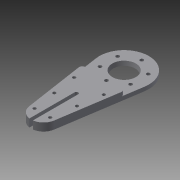
# Autodesk Inventor part: JointD0_2nd
Saved by Autodesk Inventor 2013 (Build 170138000, 138)
## iProperties
Created: 2013-02-07
Part Number: JointD0_2nd
Document SubType Name: Modeling
Designer: JohnHenry
Density: 1 g/cm^3
Material: 一般
Author: JohnHenry
Autodesk Inventor part; units mm, degrees
ref_plane "YZ Plane" through (0, 0, 0) normal (1, 0, 0) x (0, 1, 0)
ref_plane "XZ Plane" through (0, 0, 0) normal (0, 1, 0) x (-1, 0, 0)
ref_plane "XY Plane" through (0, 0, 0) normal (0, 0, 1) x (1, 0, 0)
sketch "スケッチ1" plane through (0, 0, 0) normal (0, 0, 1) x (1, 0, 0)
  circle A0 centre (0, 0) radius 15.75
  line L0 (0, -104.25) -> (0, 0)
  line L1 (0, -104.25) -> (-15.5692, -2.3795)
  line L2 (0, -104.25) -> (15.5692, -2.3795)
  point P0 (0, 15.75)
  point P1 (0, 15.75)
  dimension "d0" = 31.5
  dimension "d1" = 120
  constraints: 6 end point, 3 point on circle, 2 coincident, 2 tangent, 1 centre point, 1 vertical
  measures "d0" diameter of A0
  measures "d1" distance of L0.start A0.start
extrude "押し出し1" add sketch "スケッチ1" along normal blind 5
fillet "フィレット1" radius 8 1 edges at (0, -104.25, 2.5)
sketch "スケッチ2" plane through (0, 0, 5) normal (0, 0, 1) x (1, 0, 0)
  arc A0 (15.5692, -2.3795) -> (-15.5692, -2.3795) centre (0, 0) ccw projected
  constraints: 1 coincident
hole "Hole1" at (0, 0, 5) direction (0, 0, -1) diameter 13 depth 8 tip angle 118
sketch "スケッチ3" plane through (0, 0, 5) normal (0, 0, 1) x (1, 0, 0)
  arc A0 (-7.9082, -52.5063) -> (7.9082, -52.5063) centre (0, -51.2976) ccw projected
  line L0 (-1.1, -29.2976) -> (1.1, -29.2976)
  line L1 (1.1, -29.2976) -> (1.1, -59.2976)
  line L2 (1.1, -59.2976) -> (-1.1, -59.2976)
  line L3 (-1.1, -59.2976) -> (-1.1, -29.2976)
  dimension "d12" = 2.2
  dimension "d13" = 1.1
  dimension "d14" = 30
  dimension "d15" = 0
  constraints: 8 end point, 2 parallel, 1 horizontal, 1 perpendicular
  measures "d12" distance of L0.start L0.end
  measures "d13" distance from line of L1 A0.centre
  measures "d14" distance of L0.end L1.end
  measures "d15" distance edge to line of A0 L2
extrude "押し出し2" cut sketch "スケッチ3" against normal through all
fillet "フィレット2" radius 1 2 edges at (-1.1, -29.2976, 2.5) (1.1, -29.2976, 2.5)
sketch "スケッチ4" plane through (0, 0, 5) normal (0, 0, 1) x (1, 0, 0)
  circle A0 centre (0, 0) radius 11.25
  point P0 (0, 11.25)
  point P1 (-9.7428, 5.625)
  point P2 (-9.7428, -5.625)
  point P3 (0, -11.25)
  point P4 (9.7428, -5.625)
  point P5 (9.7428, 5.625)
  dimension "d22" = 22.5
  dimension "d25" = 360
  constraints: 1 vertical alignment, 9 other
hole "Hole2" at (0, 11.25, 5) at (-9.7428, 5.625, 5) at (-9.7428, -5.625, 5) at (0, -11.25, 5) at (9.7428, -5.625, 5) at (9.7428, 5.625, 5) direction (0, 0, -1) diameter 2.2 depth 8 tip angle 118
sketch "スケッチ5" plane through (0, 0, 5) normal (0, 0, 1) x (1, 0, 0)
  circle A0 centre (9.7428, 5.625) radius 1.1 projected
  circle A1 centre (9.7428, -5.625) radius 1.1 projected
  circle A2 centre (0, -11.25) radius 1.1 projected
  circle A3 centre (-9.7428, -5.625) radius 1.1 projected
  circle A4 centre (-9.7428, 5.625) radius 1.1 projected
  circle A5 centre (0, 11.25) radius 1.1 projected
  circle A6 centre (0, 0) radius 7.5 projected
  circle A7 centre (0, 0) radius 17
  dimension "d34" = 34
  constraints: 1 centre point
  measures "d34" diameter of A7
extrude "押し出し3" cut sketch "スケッチ5" against normal blind 2.5 contours A6 | A7
sketch "スケッチ6" plane through (0, 0, 0) normal (0, 0, -1) x (-1, 0, 0)
  circle A0 centre (-9.7428, 5.625) radius 1.1 projected
  circle A1 centre (-9.7428, -5.625) radius 1.1 projected
  circle A2 centre (0, -11.25) radius 1.1 projected
  circle A3 centre (9.7428, -5.625) radius 1.1 projected
  circle A4 centre (9.7428, 5.625) radius 1.1 projected
  circle A5 centre (0, 11.25) radius 1.1 projected
  line L0 (1.1, -30.2976) -> (1.1, -59.2216) projected
  arc A6 (1.1, -59.2216) -> (7.9082, -52.5063) centre (0, -51.2976) ccw projected
  line L1 (15.5692, -2.3795) -> (7.9082, -52.5063) projected
  arc A7 (15.5692, -2.3795) -> (-15.5692, -2.3795) centre (0, 0) ccw projected
  line L2 (-7.9082, -52.5063) -> (-15.5692, -2.3795) projected
  arc A8 (-7.9082, -52.5063) -> (-1.1, -59.2216) centre (0, -51.2976) ccw projected
  line L3 (-1.1, -59.2216) -> (-1.1, -30.2976) projected
  arc A9 (-0.1, -29.2976) -> (-1.1, -30.2976) centre (-0.1, -30.2976) ccw projected
  line L4 (-0.1, -29.2976) -> (0.1, -29.2976) projected
  arc A10 (1.1, -30.2976) -> (0.1, -29.2976) centre (0.1, -30.2976) ccw projected
  circle A11 centre (0, 0) radius 6.5 projected
extrude "押し出し4" add sketch "スケッチ6" along normal blind 2.5
chamfer "面取り2" distance 5 distance2 1 1 edges at (0, 6.5, 2.5) measured on face at (0, 6.5, 2)
sketch "スケッチ7" plane through (0, 0, -2.5) normal (0, 0, -1) x (-1, 0, 0)
  circle A0 centre (0, 0) radius 6.5 projected
  circle A1 centre (0, 11.25) radius 1.1 projected
  circle A2 centre (9.7428, 5.625) radius 1.1 projected
  circle A3 centre (9.7428, -5.625) radius 1.1 projected
  circle A4 centre (0, -11.25) radius 1.1 projected
  circle A5 centre (-9.7428, -5.625) radius 1.1 projected
  circle A6 centre (-9.7428, 5.625) radius 1.1 projected
  arc A7 (1.1, -30.2976) -> (0.1, -29.2976) centre (0.1, -30.2976) ccw projected
  line L0 (1.1, -59.2216) -> (1.1, -30.2976) projected
  arc A8 (1.1, -59.2216) -> (7.9082, -52.5063) centre (0, -51.2976) ccw projected
  line L1 (15.5692, -2.3795) -> (7.9082, -52.5063) projected
  arc A9 (15.5692, -2.3795) -> (-15.5692, -2.3795) centre (0, 0) ccw projected
  line L2 (-7.9082, -52.5063) -> (-15.5692, -2.3795) projected
  arc A10 (-7.9082, -52.5063) -> (-1.1, -59.2216) centre (0, -51.2976) ccw projected
  line L3 (-1.1, -30.2976) -> (-1.1, -59.2216) projected
  arc A11 (-0.1, -29.2976) -> (-1.1, -30.2976) centre (-0.1, -30.2976) ccw projected
  line L4 (0.1, -29.2976) -> (-0.1, -29.2976) projected
extrude "押し出し5" cut sketch "スケッチ7" against normal blind 2.5
fillet "フィレット3" radius 2 2 edges at (-14.6026, -8.7043, 3.75) (14.6026, -8.7043, 3.75)
sketch "スケッチ8" plane through (0, 0, 5) normal (0, 0, 1) x (1, 0, 0)
  line L0 (-7.9082, -52.5063) -> (-13.5882, -15.3415) projected
  line L1 (-0.1, -29.2976) -> (0.1, -29.2976) projected
  arc A0 (1.1, -59.2216) -> (7.9082, -52.5063) centre (0, -51.2976) ccw projected
  circle A1 centre (0, -51.2976) radius 5
  line L2 (-9.475, -22.3974) -> (-4.9426, -52.053)
  line L3 (0, -51.2976) -> (0, -29.2976)
  point P0 (-7.2088, -37.2252)
  point P1 (9.475, -22.3974)
  point P2 (4.9426, -52.053)
  point P3 (7.2088, -37.2252)
  dimension "d45" = 10
  dimension "d47" = 3
  dimension "d48" = 30
  constraints: 4 end point, 3 symmetric about line, 2 coincident, 2 midpoint, 1 parallel, 3 other
  measures "d47" distance from line of L0 L2.start
  measures "d48" distance of L2.start L2.end
hole "Hole3" at (-9.475, -22.3974, 5) at (-4.9426, -52.053, 5) at (-7.2088, -37.2252, 5) at (9.475, -22.3974, 5) at (7.2088, -37.2252, 5) at (4.9426, -52.053, 5) direction (0, 0, -1) diameter 2 end through all
equation "\"d13\" = 0.5 * d12"
